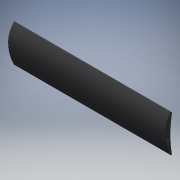
# Autodesk Inventor part: styro_50_sub
Saved by Autodesk Inventor 2018.2 (Build 222227000, 227)
## iProperties
Created: 2017-10-22
Part Number: styro_50_sub
Material: ポリスチレン
Document SubType Name: Modeling
Designer: ku_sk
Density: 1.021 g/cm^3
Appearance: カーボンファイバー
Mass: 281.605 g
Surface Area: 349.962 cm^2
Volume: 275.813 cm^3
Author: ku_sk
Autodesk Inventor part; units mm, degrees
ref_plane "YZ Plane" through (0, 0, 0) normal (1, 0, 0) x (0, 1, 0)
ref_plane "XZ Plane" through (0, 0, 0) normal (0, 1, 0) x (-1, 0, 0)
ref_plane "XY Plane" through (0, 0, 0) normal (0, 0, 1) x (1, 0, 0)
sketch "スケッチ1" plane through (0, 0, 0) normal (1, 0, 0) x (0, 1, 0)
  line L0 (0, 125) -> (0, -125)
  line L1 (-193.7075, 0) -> (764.5712, 0) projected
  arc A0 (0, 125) -> (0, -125) centre (627.6743, 0) ccw
  arc A1 (0, 125) -> (-45.1737, 25) centre (79.0119, 29.1041) ccw
  arc A2 (-45.1737, 25) -> (0, -125) centre (259.9333, 35.0832) ccw
  point P0 (0, 0)
  point P1 (0, 0)
  dimension "d0" = 250
  dimension "d1" = 640
  dimension "d16" = 100
  constraints: 6 point on circle, 3 centre point, 2 end point, 2 midpoint, 1 point on line, 1 tangent, 1 vertical
  measures "d0" distance of L0.start L0.end
  measures "d1" radius of A0
  measures "d16" vertical distance of A1.end L0.start
extrude "押し出し4" add sketch "スケッチ1" along normal mid plane 950 contours A0 L1 A2 A1 | A0 A2 L1
fillet "フィレット3" radius 5 1 edges at (0, 0, 125)
fillet "フィレット3" radius 3 1 edges at (0, 0, -125)
sketch "スケッチ4" plane through (475, 0, 0) normal (1, 0, 0) x (0, 0, -1)
  circle A0 centre (23.3804, -26.1259) radius 6
  arc A1 (109.8042, -8.7665) -> (107.8747, -3.1688) centre (108.3804, -6.1259) ccw projected
  point P0 (0, 0)
  dimension "d21" = 12
  dimension "d22" = 85
  dimension "d23" = 20
  constraints: 1 centre point
  measures "d21" diameter of A0
  measures "d22" horizontal distance of A1.centre A0.centre
  measures "d23" vertical distance of A1.centre A0.centre
extrude "押し出し5" cut sketch "スケッチ4" against normal through all
